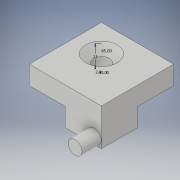
# Autodesk Inventor part: Door pin right
Saved by Autodesk Inventor 2019 (Build 230136000, 136)
## iProperties
Created: 2019-02-11
Part Number: Door pin right
Material: Generic
Document SubType Name: Modeling
Designer: aonih
Density: 1 g/cm^3
Appearance: Default
Author: aonih
Autodesk Inventor part; units mm, degrees
ref_plane "YZ Plane" through (0, 0, 0) normal (1, 0, 0) x (0, 1, 0)
ref_plane "XZ Plane" through (0, 0, 0) normal (0, 1, 0) x (-1, 0, 0)
ref_plane "XY Plane" through (0, 0, 0) normal (0, 0, 1) x (1, 0, 0)
sketch "Sketch2" plane through (0, 0, 0) normal (0, 1, 0) x (-1, 0, 0)
  line L0 (12.7, 12.7) -> (-12.7, 12.7)
  line L1 (-12.7, 12.7) -> (-12.7, -12.7)
  line L2 (-12.7, -12.7) -> (12.7, -12.7)
  line L3 (12.7, -12.7) -> (12.7, 12.7)
  line L4 (12.7, 0) -> (-12.7, 0) construction
  line L5 (0, -12.7) -> (0, 12.7) construction
  point P0 (0, 0)
  point P1 (0, 0)
  dimension "d2" = 25.4
  dimension "d3" = 25.4
  constraints: 12 end point, 5 midpoint, 2 parallel, 1 coincident, 1 horizontal, 1 perpendicular
  measures "d2" distance of L2.end L0.start
  measures "d3" distance of L1.end L2.end
extrude "Base" add sketch "Sketch2" against normal blind 6.5
sketch "Sketch3" plane through (0, -6.5, 0) normal (0, -1, 0) x (1, 0, 0)
  line L0 (12.7, 12.7) -> (-12.7, 12.7) projected
  line L1 (12.7, 12.7) -> (6.35, 12.7)
  line L2 (6.35, 12.7) -> (6.35, 0)
  line L3 (6.35, 0) -> (12.7, 0)
  line L4 (12.7, 0) -> (12.7, 12.7)
  line L5 (0, 12.7) -> (6.35, 12.7)
  line L6 (6.35, 12.7) -> (6.35, 6.35)
  line L7 (6.35, 6.35) -> (0, 6.35)
  line L8 (0, 6.35) -> (0, 12.7)
  line L9 (-12.7, 12.7) -> (-12.7, -12.7) projected
  line L10 (12.7, 12.7) -> (-12.7, 12.7)
  line L11 (-12.7, 12.7) -> (-12.7, -12.7)
  line L12 (-12.7, -12.7) -> (12.7, -12.7)
  line L13 (12.7, -12.7) -> (12.7, 12.7)
  point P0 (0, 0)
  dimension "d6" = 6.35
  dimension "d7" = 12.7
  constraints: 24 end point, 6 parallel, 3 horizontal, 3 perpendicular, 2 midpoint
  measures "d6" distance of L3.end L2.end
  measures "d7" distance of L3.end L0.start
extrude "Back extrusion" add sketch "Sketch3" along normal blind 6.5 contours L4 L3 L2 L0 | L2 L7 L8 L0
sketch "Sketch5" plane through (-12.7, 0, 12.7) normal (0, 0, 1) x (1, 0, 0)
  line L0 (12.7, -6.5) -> (0, -6.5) projected
  line L1 (25.4, -6.5) -> (25.4, -13) projected
  line L2 (12.7, -6.5) -> (25.4, -6.5) construction
  line L3 (25.4, -13) -> (12.7, -13) projected
  line L4 (25.4, -13) -> (20.4, -13) construction
  line L5 (20.4, -13) -> (20.4, -8) construction
  line L6 (20.4, -8) -> (25.4, -8) construction
  line L7 (25.4, -8) -> (25.4, -13) construction
  line L8 (20.4, -8) -> (25.4, -13) construction
  line L9 (20.4, -13) -> (25.4, -8) construction
  circle A0 centre (22.9, -10.5) radius 2.425
  point P0 (12.7, 0)
  dimension "d10" = 5
  dimension "d11" = 5
  dimension "d12" = 4.85
  constraints: 14 end point, 2 horizontal, 2 parallel, 1 centre point, 1 midpoint, 1 perpendicular
  measures "d10" distance of L5.end L6.end
  measures "d11" distance of L4.end L5.end
  measures "d12" diameter of A0
extrude "Extrusion3" add sketch "Sketch5" along normal blind 6.75
sketch "Sketch6" plane through (0, -6.5, 0) normal (0, -1, 0) x (1, 0, 0)
  line L0 (-12.7, 12.7) -> (-12.7, -12.7) projected
  line L1 (-12.7, -12.7) -> (-4.9218, -4.9218) construction
  line L2 (-12.7, -12.7) -> (-1.7, -12.7) construction
  line L3 (-4.9218, -4.9218) -> (-3.1541, -3.1541) construction
  line L4 (-4.9218, -4.9218) -> (-2.4218, -4.9218) construction
  circle A0 centre (-3.1541, -3.1541) radius 2.5
  point P0 (0, 0)
  dimension "d15" = 11
  dimension "d16" = 45
  dimension "d17" = 2.5
  dimension "d18" = 45
  constraints: 8 end point, 2 equal length, 2 horizontal, 1 coincident, 3 other
  measures "d15" distance of L0.end L1.end
  measures "d16" angle of L2 L1
  measures "d17" distance of L1.end L3.end
  measures "d18" angle of L4 L3
sketch "Sketch7" plane through (0, 0, 0) normal (0, 1, 0) x (1, 0, 0)
  line L0 (-12.7, -12.7) -> (-12.7, 12.7) projected
  line L1 (-12.7, 12.7) -> (-7.0431, 7.0431) construction
  line L2 (-12.7, 12.7) -> (-4.7, 12.7) construction
  line L3 (-7.0431, 7.0431) -> (-3.1541, 3.1541) construction
  line L4 (-7.0431, 7.0431) -> (-1.5431, 7.0431) construction
  circle A0 centre (-3.1541, 3.1541) radius 5.5
  point P0 (0, 0)
  dimension "d19" = 8
  dimension "d20" = 45
  dimension "d21" = 5.5
  dimension "d22" = 45
  constraints: 8 end point, 2 equal length, 2 horizontal, 1 coincident, 3 other
  measures "d19" distance of L0.end L1.end
  measures "d20" angle of L1 L2
  measures "d21" distance of L1.end L3.end
  measures "d22" angle of L3 L4
hole "Hole1" at (-3.1541, 0, -3.1541) direction (0, -1, 0) diameter 5.5 end through all countersink diameter 11 countersink angle 90
equation "\"d3\" = d2"
equation "\"d7\" = 2 * d6"
equation "\"d11\" = d10"
body "Solid1"
